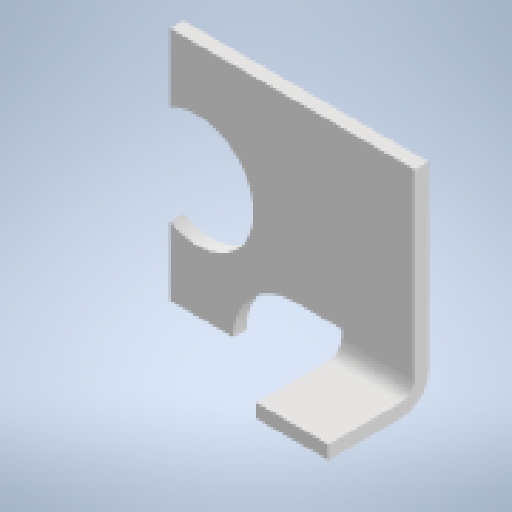
# Autodesk Inventor part: hipjoint_toleg_under_up_right
Saved by Autodesk Inventor 2024.1 (Build 281209000, 209)
## iProperties
Created: 2024-10-09
Part Number: hipjoint_toleg_under_up_right
Material: 一般
Document SubType Name: Sheet Metal
Designer: hibik
Density: 1 g/cm^3
Sheet Metal Rule: Default_mm
Appearance: 既定
Author: hibik
Autodesk Inventor part; units mm, degrees
ref_plane "YZ Plane" through (0, 0, 0) normal (1, 0, 0) x (0, 1, 0)
ref_plane "XZ Plane" through (0, 0, 0) normal (0, 1, 0) x (-1, 0, 0)
ref_plane "XY Plane" through (0, 0, 0) normal (0, 0, 1) x (1, 0, 0)
sketch "スケッチ1" plane through (0, 0, 0) normal (0, 0, 1) x (1, 0, 0)
  circle A0 centre (0, 0) radius 6.25
  line L0 (0, 13) -> (24, 13)
  line L1 (24, 13) -> (24, -13)
  line L2 (24, -13) -> (0, -13)
  line L3 (0, -13) -> (0, 13)
  line L4 (0, 13) -> (-3, 13)
  line L5 (-3, 13) -> (-3, -13)
  line L6 (-3, -13) -> (0, -13)
  line L7 (0, -13) -> (0, 13)
  line L8 (16, -13) -> (16, -6.25)
  line L9 (16, -6.25) -> (0, -6.25)
  line L10 (-3, -10) -> (24, -10)
  arc A1 (10.75, -6.25) -> (4, -13) centre (10.75, -13) ccw
  line L11 (4, -13) -> (4, -9.651) construction
  point P0 (24, 0)
  point P1 (-3, 5.4829)
  point P2 (-3, -5.4829)
  point P3 (0, 0)
  point P4 (16, -10)
  point P5 (4.7033, -10)
  dimension "d0" = 12.5
  dimension "d1" = 24
  dimension "d2" = 26
  dimension "d3" = 3
  dimension "d5" = 8
  dimension "d16" = 3
  dimension "d17" = 7
  measures "d1" distance of L1.end L2.end
  measures "d2" distance of L0.end L1.end
  measures "d3" distance of L6.end L5.end
  measures "d5" distance between parallel lines of L1 L8
  measures "d16" distance between parallel lines of L10 L2
  measures "d17" distance between parallel lines of L11 L5
extrude "プレート1" add sketch "スケッチ1" along normal blind 1.5 contours L3 L10 L5 A0 | L9 A1 L10 L3 | A0 L3 L0 L1 L10 L8 L9 | L10 A1 L2 L3 | L3 L6 L5 L10 | A0 L5 L4 L3
sketch "スケッチ2" plane through (24, -8.5, 0) normal (0, -1, 0) x (1, 0, 0)
  line L0 (-8, 0) -> (0, 0)
  line L1 (0, 0) -> (0, 11)
  line L2 (0, 11) -> (-8, 11)
  line L3 (-8, 11) -> (-8, 0)
  constraints: 6 end point, 1 horizontal, 1 perpendicular, 1 vertical
edge flange "フランジ1" height 11 angle 90 thickness 1.5 bend radius 1.5 thickness toward (0, -1, 0) relief tear relief width 1.5 relief depth 0.75 edges at (20, -10, 1.5) wall of the first edge with corners at (16, -8.5, 0) (24, -8.5, 0) (24, -8.5, 11) (16, -8.5, 11)
bend "曲げ1"
corner "コーナー1"
equation "\"d4\" = Thickness"
equation "\"d6\" = BendReliefWidth"
equation "\"d7\" = BendReliefDepth"
equation "\"d8\" = MinimumRemnant"
equation "\"d9\" = TransitionRadius"
equation "\"d12\" = BendRadius"
equation "\"d13\" = CornerReliefSize"
equation "\"d14\" = GapSize"
equation "\"d15\" = JacobiRadiusSize"
equation "\"BendRadius\" = Thickness"
equation "\"BendReliefWidth\" = Thickness"
equation "\"BendReliefDepth\" = 0.5 * Thickness"
equation "\"CornerReliefSize\" = 4 * Thickness"
equation "\"MinimumRemnant\" = 2 * Thickness"
equation "\"TransitionRadius\" = BendRadius"
equation "\"JacobiRadiusSize\" = BendRadius"
equation "\"GapSize\" = Thickness"
equation "\"Thickness\" = 1.5"
